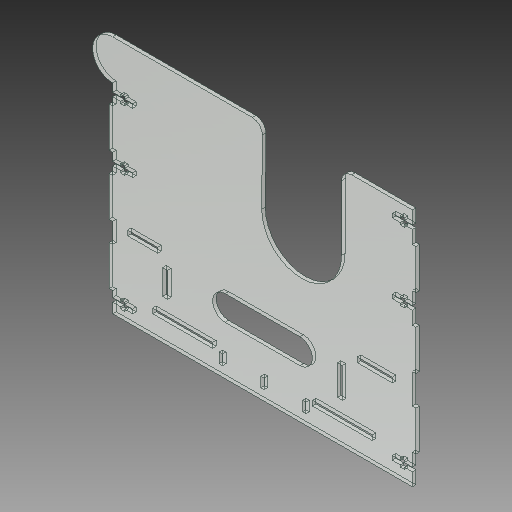
# Autodesk Inventor part: Lat_Der_Caja
Saved by Autodesk Inventor 2019 (Build 230136000, 136)
## iProperties
Created: 2020-04-06
Part Number: Lat_Der_Caja
Material: Generic
Document SubType Name: Modeling
Designer: Jurgen
Density: 1 g/cm^3
Appearance: Clear
Author: Jurgen
Autodesk Inventor part; units mm, degrees
ref_plane "YZ Plane" through (0, 0, 0) normal (1, 0, 0) x (0, 1, 0)
ref_plane "XZ Plane" through (0, 0, 0) normal (0, 1, 0) x (-1, 0, 0)
ref_plane "XY Plane" through (0, 0, 0) normal (0, 0, 1) x (1, 0, 0)
sketch "Sketch1" plane through (0, 0, 0) normal (0, 0, 1) x (1, 0, 0)
  line L0 (0.3285, -0.1681) -> (0.3285, -5.1681)
  line L1 (60.3285, -5.1681) -> (0.3285, -5.1681)
  line L2 (60.3285, -0.1681) -> (60.3285, -5.1681)
  line L3 (0.3285, -0.1681) -> (60.3285, -0.1681)
  line L4 (15.3285, 39.8319) -> (15.3285, 14.8319)
  line L5 (15.3285, 14.8319) -> (10.3285, 14.8319)
  line L6 (10.3285, 14.8319) -> (10.3285, 39.8319)
  line L7 (15.3285, 39.8319) -> (10.3285, 39.8319)
  line L8 (-24.6715, 54.8319) -> (-24.6715, 49.8319)
  line L9 (-24.6715, 54.8319) -> (5.3285, 54.8319)
  line L10 (5.3285, 49.8319) -> (-24.6715, 49.8319)
  line L11 (5.3285, 54.8319) -> (5.3285, 49.8319)
  line L12 (220.3285, -5.1681) -> (160.3285, -5.1681)
  line L13 (160.3285, -0.1681) -> (160.3285, -5.1681)
  line L14 (160.3285, -0.1681) -> (220.3285, -0.1681)
  line L15 (220.3285, -0.1681) -> (220.3285, -5.1681)
  line L16 (190.3285, 14.8319) -> (185.3285, 14.8319)
  line L17 (185.3285, 14.8319) -> (185.3285, 44.8319)
  line L18 (190.3285, 44.8319) -> (190.3285, 14.8319)
  line L19 (190.3285, 44.8319) -> (185.3285, 44.8319)
  line L20 (205.3285, 59.8319) -> (205.3285, 54.8319)
  line L21 (240.3285, 59.8319) -> (205.3285, 59.8319)
  line L22 (240.3285, 54.8319) -> (205.3285, 54.8319)
  line L23 (240.3285, 59.8319) -> (240.3285, 54.8319)
  line L24 (260.3283, -5.1682) -> (260.3283, 214.8318) construction
  line L25 (260.3283, 214.8318) -> (230.3283, 214.8318) construction
  circle A0 centre (149.5, 140) radius 18.5 construction
  circle A1 centre (149.5, 140) radius 12.5 construction
  arc A2 (132.0393, 133.8144) -> (122.7954, 140) centre (122.7954, 130) ccw construction
  arc A3 (134.5683, 127.6856) -> (143.8122, 121.5) centre (143.8122, 131.5) ccw construction
  line L26 (132.0393, 133.8144) -> (134.5683, 127.6856) construction
  line L27 (143.8122, 121.5) -> (185.1878, 121.5) construction
  arc A4 (185.1878, 121.5) -> (194.4317, 127.6856) centre (185.1878, 131.5) ccw construction
  line L28 (194.4317, 127.6856) -> (196.9607, 133.8144) construction
  arc A5 (206.2046, 140) -> (196.9607, 133.8144) centre (206.2046, 130) ccw construction
  line L29 (206.2046, 140) -> (250, 140) construction
  line L30 (81.6779, 140) -> (122.7954, 140) construction
  line L31 (-39.6717, -25.1682) -> (260.3283, -25.1682)
  line L32 (260.3283, -25.1682) -> (260.3283, 214.8318)
  circle A6 centre (149.5, 140) radius 40 construction
  line L33 (-39.6717, 214.8318) -> (-39.6717, -25.1682)
  line L34 (-39.6717, 214.8318) -> (80.3283, 214.8318)
  line L35 (260.3283, 214.8318) -> (-39.6717, 214.8318) construction
  line L36 (215.3283, 214.8318) -> (260.3283, 214.8318) construction
  line L37 (215.3283, 214.8318) -> (260.3283, 214.8318)
  line L38 (109.5, 140) -> (189.5, 140) construction
  arc A7 (109.5, 140) -> (189.5, 140) centre (149.5, 140) ccw
  line L39 (109.5, 140) -> (110.3283, 214.8318)
  line L40 (110.3283, 214.8318) -> (80.3283, 214.8318)
  line L41 (189.5, 140) -> (189.5, 214.8318)
  line L42 (189.5, 214.8318) -> (215.3283, 214.8318)
  line L43 (0.3283, -25.1682) -> (0.3283, 214.8318) construction
  point P0 (0, 0)
  point P1 (113.145, 123.3174)
  point P2 (184.723, 121.0438)
  dimension "d0" = 300
  dimension "d1" = 220
  dimension "d2" = 80
  dimension "d3" = 240
  dimension "d6" = 45
  dimension "d84" = 40
  constraints: 88 end point, 14 point on circle, 8 centre point, 6 horizontal, 5 point on line, 4 vertical, 3 collinear, 2 perpendicular, 1 coincident, 1 concentric, 1 midpoint, 19 other
  measures "d0" distance of L33.start L24.end
  measures "d1" distance of L24.start L24.end
  measures "d2" diameter of A6
  measures "d3" distance of L33.start L31.start
  measures "d6" distance of L24.end L36.start
  measures "d84" distance between parallel lines of L33 L43
extrude "Extrusion1" add sketch "Sketch1" along normal blind 3.5
fillet "Fillet1" radius 10 2 edges at (110.3283, 214.8318, 1.75) (189.5, 214.8318, 1.75)
sketch "Sketch3" plane through (0, 0, 3.5) normal (0, 0, 1) x (1, 0, 0)
  arc A0 (199.5, 214.8318) -> (189.5, 204.8318) centre (199.5, 204.8318) ccw construction
  line L0 (189.5, 204.8318) -> (189.5, 140) construction
  arc A1 (109.5, 140) -> (189.5, 140) centre (149.5, 140) ccw construction
  line L1 (109.5, 140) -> (110.2164, 204.7211) construction
  arc A2 (110.2164, 204.7211) -> (100.217, 214.8318) centre (100.217, 204.8318) ccw construction
  line L2 (100.217, 214.8318) -> (-39.6717, 214.8318) construction
  line L3 (-39.6717, 214.8318) -> (-39.6717, -25.1682) construction
  line L4 (-39.6717, -25.1682) -> (260.3283, -25.1682) construction
  line L5 (260.3283, -25.1682) -> (260.3283, 214.8318) construction
  line L6 (260.3283, 214.8318) -> (199.5, 214.8318) construction
  line L7 (160.3285, -5.1681) -> (160.3285, -0.1681) construction
  line L8 (160.3285, -0.1681) -> (220.3285, -0.1681) construction
  line L9 (220.3285, -0.1681) -> (220.3285, -5.1681) construction
  line L10 (220.3285, -5.1681) -> (160.3285, -5.1681) construction
  line L11 (0.3285, -0.1681) -> (60.3285, -0.1681) construction
  line L12 (60.3285, -0.1681) -> (60.3285, -5.1681) construction
  line L13 (60.3285, -5.1681) -> (0.3285, -5.1681) construction
  line L14 (0.3285, -5.1681) -> (0.3285, -0.1681) construction
  line L15 (205.3285, 59.8319) -> (240.3285, 59.8319) construction
  line L16 (240.3285, 59.8319) -> (240.3285, 54.8319) construction
  line L17 (240.3285, 54.8319) -> (205.3285, 54.8319) construction
  line L18 (205.3285, 54.8319) -> (205.3285, 59.8319) construction
  line L19 (185.3285, 14.8319) -> (185.3285, 44.8319) construction
  line L20 (185.3285, 44.8319) -> (190.3285, 44.8319) construction
  line L21 (190.3285, 44.8319) -> (190.3285, 14.8319) construction
  line L22 (190.3285, 14.8319) -> (185.3285, 14.8319) construction
  line L23 (-24.6715, 54.8319) -> (5.3285, 54.8319) construction
  line L24 (5.3285, 54.8319) -> (5.3285, 49.8319) construction
  line L25 (5.3285, 49.8319) -> (-24.6715, 49.8319) construction
  line L26 (-24.6715, 49.8319) -> (-24.6715, 54.8319) construction
  line L27 (15.3285, 14.8319) -> (10.3285, 14.8319) construction
  line L28 (10.3285, 14.8319) -> (10.3285, 39.8319) construction
  line L29 (10.3285, 39.8319) -> (15.3285, 39.8319) construction
  line L30 (15.3285, 39.8319) -> (15.3285, 14.8319) construction
  line L31 (-39.6717, 214.8318) -> (-39.6717, -25.1682) construction
  arc A3 (-39.6717, 174.8318) -> (-50.6681, 178.1261) centre (-39.6717, 194.8318) ccw construction
  arc A4 (-39.6717, 214.8318) -> (-50.6681, 178.1261) centre (-39.6717, 194.8318) ccw
  line L32 (-39.6717, 174.8318) -> (-39.6717, 159.8318)
  line L33 (-39.6717, 174.8318) -> (-39.6717, 214.8318)
  line L34 (-39.6717, 94.8318) -> (-43.1717, 94.8318)
  line L35 (-43.1717, 94.8318) -> (-43.1717, 54.8318)
  line L36 (-43.1717, 54.8318) -> (-39.6717, 54.8318)
  line L37 (-39.6717, 54.8318) -> (-39.6717, 94.8318)
  line L38 (-39.6717, -5.1682) -> (-43.1717, -5.1682)
  line L39 (-43.1717, -5.1682) -> (-43.1717, 34.8318)
  line L40 (-43.1717, 34.8318) -> (-39.6717, 34.8318)
  line L41 (-39.6717, 34.8318) -> (-39.6717, -5.1682)
  line L42 (-39.6717, 154.8318) -> (-43.1717, 154.8318)
  line L43 (-43.1717, 154.8318) -> (-43.1717, 114.8318)
  line L44 (-43.1717, 114.8318) -> (-39.6717, 114.8318)
  line L45 (-39.6717, 114.8318) -> (-39.6717, 154.8318)
  line L46 (-39.6717, -25.1682) -> (-39.6717, 214.8318) construction
  line L47 (110.3283, -25.1682) -> (110.3283, 54.8318) construction
  line L48 (260.3283, 184.8318) -> (263.8283, 184.8318)
  line L49 (263.8283, 184.8318) -> (263.8283, 144.8318)
  line L50 (263.8283, 144.8318) -> (260.3283, 144.8318)
  line L51 (260.3283, 144.8318) -> (260.3283, 184.8318)
  line L52 (260.3283, -25.1682) -> (260.3283, 214.8318) construction
  line L53 (260.3283, 114.8318) -> (263.8283, 114.8318)
  line L54 (263.8283, 114.8318) -> (263.8283, 74.8318)
  line L55 (263.8283, 74.8318) -> (260.3283, 74.8318)
  line L56 (260.3283, 74.8318) -> (260.3283, 114.8318)
  line L57 (260.3283, 44.8318) -> (263.8283, 44.8318)
  line L58 (263.8283, 44.8318) -> (263.8283, 4.8318)
  line L59 (263.8283, 4.8318) -> (260.3283, 4.8318)
  line L60 (260.3283, 4.8318) -> (260.3283, 44.8318)
  arc A5 (-39.6717, 214.8318) -> (-39.6717, 174.8318) centre (-39.6717, 194.8318) ccw
  point P0 (0, 0)
  dimension "d21" = 40
  dimension "d22" = 20
  dimension "d23" = 15
  dimension "d24" = 3.5
  dimension "d25" = 40
  dimension "d26" = 3.5
  dimension "d27" = 40
  dimension "d28" = 20
  dimension "d29" = 20
  dimension "d30" = 3.5
  dimension "d31" = 40
  dimension "d32" = 20
  dimension "d35" = 3.5
  dimension "d36" = 40
  dimension "d37" = 3.5
  dimension "d38" = 40
  dimension "d39" = 3.5
  dimension "d40" = 40
  dimension "d41" = 30
  dimension "d42" = 30
  dimension "d43" = 30
  constraints: 56 end point, 12 parallel, 8 point on line, 6 horizontal, 6 perpendicular, 6 point on circle, 3 centre point, 3 tangent, 1 midpoint, 1 vertical
  measures "d21" diameter of A3
  measures "d22" distance from line of L2 A3.centre
  measures "d23" distance of L32.start L32.end
  measures "d24" distance of L36.end L35.end
  measures "d25" distance of L35.end L34.end
  measures "d26" distance of L39.end L40.end
  measures "d27" distance of L38.end L39.end
  measures "d28" distance between parallel lines of L4 L38
  measures "d29" distance between parallel lines of L40 L36
  measures "d30" distance of L44.end L43.end
  measures "d31" distance of L43.end L42.end
  measures "d32" distance from line of L34.end L44
  measures "d35" distance of L49.end L50.end
  measures "d36" distance of L48.end L49.end
  measures "d37" distance of L54.end L55.end
  measures "d38" distance of L53.end L54.end
  measures "d39" distance of L58.end L59.end
  measures "d40" distance of L57.end L58.end
  measures "d41" distance between parallel lines of L4 L59
  measures "d42" distance between parallel lines of L57 L55
  measures "d43" distance between parallel lines of L53 L50
extrude "Extrusion3" add sketch "Sketch3" against normal blind 3.5
sketch "Sketch4" plane through (0, 0, 3.5) normal (0, 0, 1) x (1, 0, 0)
  arc A0 (199.5, 214.8318) -> (189.5, 204.8318) centre (199.5, 204.8318) ccw construction
  line L0 (189.5, 204.8318) -> (189.5, 140) construction
  arc A1 (109.5, 140) -> (189.5, 140) centre (149.5, 140) ccw construction
  line L1 (109.5, 140) -> (110.2164, 204.7211) construction
  arc A2 (110.2164, 204.7211) -> (100.217, 214.8318) centre (100.217, 204.8318) ccw construction
  line L2 (100.217, 214.8318) -> (-39.6717, 214.8318) construction
  arc A3 (-39.6717, 214.8318) -> (-39.6717, 174.8318) centre (-39.6717, 194.8318) ccw construction
  line L3 (-39.6717, 174.8318) -> (-39.6717, 154.8318) construction
  line L4 (-39.6717, 154.8318) -> (-43.1717, 154.8318) construction
  line L5 (-43.1717, 154.8318) -> (-43.1717, 114.8318) construction
  line L6 (-43.1717, 114.8318) -> (-39.6717, 114.8318) construction
  line L7 (-39.6717, 114.8318) -> (-39.6717, 94.8318) construction
  line L8 (-39.6717, 94.8318) -> (-43.1717, 94.8318) construction
  line L9 (-43.1717, 94.8318) -> (-43.1717, 54.8318) construction
  line L10 (-43.1717, 54.8318) -> (-39.6717, 54.8318) construction
  line L11 (-39.6717, 54.8318) -> (-39.6717, 34.8318) construction
  line L12 (-43.1717, 34.8318) -> (-39.6717, 34.8318) construction
  line L13 (-43.1717, -5.1682) -> (-43.1717, 34.8318) construction
  line L14 (-39.6717, -5.1682) -> (-43.1717, -5.1682) construction
  line L15 (-39.6717, -5.1682) -> (-39.6717, -25.1682) construction
  line L16 (-39.6717, -25.1682) -> (260.3283, -25.1682) construction
  line L17 (260.3283, -25.1682) -> (260.3283, 4.8318) construction
  line L18 (263.8283, 4.8318) -> (260.3283, 4.8318) construction
  line L19 (263.8283, 44.8318) -> (263.8283, 4.8318) construction
  line L20 (260.3283, 44.8318) -> (263.8283, 44.8318) construction
  line L21 (260.3283, 44.8318) -> (260.3283, 74.8318) construction
  line L22 (263.8283, 74.8318) -> (260.3283, 74.8318) construction
  line L23 (263.8283, 114.8318) -> (263.8283, 74.8318) construction
  line L24 (260.3283, 114.8318) -> (263.8283, 114.8318) construction
  line L25 (260.3283, 114.8318) -> (260.3283, 144.8318) construction
  line L26 (263.8283, 144.8318) -> (260.3283, 144.8318) construction
  line L27 (263.8283, 184.8318) -> (263.8283, 144.8318) construction
  line L28 (260.3283, 184.8318) -> (263.8283, 184.8318) construction
  line L29 (260.3283, 184.8318) -> (260.3283, 214.8318) construction
  line L30 (260.3283, 214.8318) -> (199.5, 214.8318) construction
  line L31 (160.3285, -5.1681) -> (160.3285, -0.1681) construction
  line L32 (160.3285, -0.1681) -> (220.3285, -0.1681) construction
  line L33 (220.3285, -0.1681) -> (220.3285, -5.1681) construction
  line L34 (220.3285, -5.1681) -> (160.3285, -5.1681) construction
  line L35 (0.3285, -0.1681) -> (60.3285, -0.1681) construction
  line L36 (60.3285, -0.1681) -> (60.3285, -5.1681) construction
  line L37 (60.3285, -5.1681) -> (0.3285, -5.1681) construction
  line L38 (0.3285, -5.1681) -> (0.3285, -0.1681) construction
  line L39 (205.3285, 59.8319) -> (240.3285, 59.8319) construction
  line L40 (240.3285, 59.8319) -> (240.3285, 54.8319) construction
  line L41 (240.3285, 54.8319) -> (205.3285, 54.8319) construction
  line L42 (205.3285, 54.8319) -> (205.3285, 59.8319) construction
  line L43 (185.3285, 14.8319) -> (185.3285, 44.8319) construction
  line L44 (185.3285, 44.8319) -> (190.3285, 44.8319) construction
  line L45 (190.3285, 44.8319) -> (190.3285, 14.8319) construction
  line L46 (190.3285, 14.8319) -> (185.3285, 14.8319) construction
  line L47 (-24.6715, 54.8319) -> (5.3285, 54.8319) construction
  line L48 (5.3285, 54.8319) -> (5.3285, 49.8319) construction
  line L49 (5.3285, 49.8319) -> (-24.6715, 49.8319) construction
  line L50 (-24.6715, 49.8319) -> (-24.6715, 54.8319) construction
  line L51 (15.3285, 14.8319) -> (10.3285, 14.8319) construction
  line L52 (10.3285, 14.8319) -> (10.3285, 39.8319) construction
  line L53 (10.3285, 39.8319) -> (15.3285, 39.8319) construction
  line L54 (15.3285, 39.8319) -> (15.3285, 14.8319) construction
  line L55 (-39.6717, 174.8318) -> (-39.6717, 154.8318) construction
  line L56 (-39.6717, 162.8318) -> (-19.6717, 162.8318) construction
  line L57 (-19.6717, 162.8318) -> (-19.6717, 166.8318) construction
  line L58 (-19.6717, 166.8318) -> (-39.6717, 166.8318) construction
  line L59 (-39.6717, 166.8318) -> (-39.6717, 162.8318) construction
  line L60 (-39.6717, 164.8318) -> (-19.6717, 164.8318) construction
  line L61 (-31.6717, 160.8318) -> (-27.6717, 160.8318) construction
  line L62 (-27.6717, 160.8318) -> (-27.6717, 168.8318) construction
  line L63 (-27.6717, 168.8318) -> (-31.6717, 168.8318) construction
  line L64 (-31.6717, 168.8318) -> (-31.6717, 160.8318) construction
  line L65 (-31.6717, 160.8318) -> (-27.6717, 168.8318) construction
  line L66 (-27.6717, 160.8318) -> (-31.6717, 168.8318) construction
  line L67 (-39.6717, 166.8318) -> (-39.6717, 162.8318)
  line L68 (-39.6717, 162.8318) -> (-31.6717, 162.8318)
  line L69 (-31.6717, 162.8318) -> (-31.6717, 160.8318)
  line L70 (-31.6717, 160.8318) -> (-27.6717, 160.8318)
  line L71 (-27.6717, 160.8318) -> (-27.6717, 162.8318)
  line L72 (-27.6717, 162.8318) -> (-19.6717, 162.8318)
  line L73 (-19.6717, 162.8318) -> (-19.6717, 166.8318)
  line L74 (-19.6717, 166.8318) -> (-27.6717, 166.8318)
  line L75 (-27.6717, 166.8318) -> (-27.6717, 168.8318)
  line L76 (-27.6717, 168.8318) -> (-31.6717, 168.8318)
  line L77 (-31.6717, 168.8318) -> (-31.6717, 166.8318)
  line L78 (-31.6717, 166.8318) -> (-39.6717, 166.8318)
  line L79 (-39.6717, 102.8318) -> (-19.6717, 102.8318) construction
  line L80 (-19.6717, 102.8318) -> (-19.6717, 106.8318) construction
  line L81 (-19.6717, 106.8318) -> (-39.6717, 106.8318) construction
  line L82 (-39.6717, 106.8318) -> (-39.6717, 102.8318) construction
  line L83 (-39.6717, 104.8318) -> (-19.6717, 104.8318) construction
  line L84 (-31.6717, 100.8318) -> (-27.6717, 100.8318) construction
  line L85 (-27.6717, 100.8318) -> (-27.6717, 108.8318) construction
  line L86 (-27.6717, 108.8318) -> (-31.6717, 108.8318) construction
  line L87 (-31.6717, 108.8318) -> (-31.6717, 100.8318) construction
  line L88 (-31.6717, 100.8318) -> (-27.6717, 108.8318) construction
  line L89 (-27.6717, 100.8318) -> (-31.6717, 108.8318) construction
  line L90 (-39.6717, 106.8318) -> (-39.6717, 102.8318)
  line L91 (-39.6717, 102.8318) -> (-31.6717, 102.8318)
  line L92 (-31.6717, 102.8318) -> (-31.6717, 100.8318)
  line L93 (-31.6717, 100.8318) -> (-27.6717, 100.8318)
  line L94 (-27.6717, 100.8318) -> (-27.6717, 102.8318)
  line L95 (-27.6717, 102.8318) -> (-19.6717, 102.8318)
  line L96 (-19.6717, 102.8318) -> (-19.6717, 106.8318)
  line L97 (-19.6717, 106.8318) -> (-27.6717, 106.8318)
  line L98 (-27.6717, 106.8318) -> (-27.6717, 108.8318)
  line L99 (-27.6717, 108.8318) -> (-31.6717, 108.8318)
  line L100 (-31.6717, 108.8318) -> (-31.6717, 106.8318)
  line L101 (-31.6717, 106.8318) -> (-39.6717, 106.8318)
  line L102 (-39.6717, -15.1682) -> (-19.6717, -15.1682) construction
  line L103 (-19.6717, -15.1682) -> (-19.6717, -11.1682) construction
  line L104 (-19.6717, -11.1682) -> (-39.6717, -11.1682) construction
  line L105 (-39.6717, -11.1682) -> (-39.6717, -15.1682) construction
  line L106 (-39.6717, -13.1682) -> (-19.6717, -13.1682) construction
  line L107 (-31.6717, -17.1682) -> (-27.6717, -17.1682) construction
  line L108 (-27.6717, -17.1682) -> (-27.6717, -9.1682) construction
  line L109 (-27.6717, -9.1682) -> (-31.6717, -9.1682) construction
  line L110 (-31.6717, -9.1682) -> (-31.6717, -17.1682) construction
  line L111 (-31.6717, -17.1682) -> (-27.6717, -9.1682) construction
  line L112 (-27.6717, -17.1682) -> (-31.6717, -9.1682) construction
  line L113 (-39.6717, -11.1682) -> (-39.6717, -15.1682)
  line L114 (-39.6717, -15.1682) -> (-31.6717, -15.1682)
  line L115 (-31.6717, -15.1682) -> (-31.6717, -17.1682)
  line L116 (-31.6717, -17.1682) -> (-27.6717, -17.1682)
  line L117 (-27.6717, -17.1682) -> (-27.6717, -15.1682)
  line L118 (-27.6717, -15.1682) -> (-19.6717, -15.1682)
  line L119 (-19.6717, -15.1682) -> (-19.6717, -11.1682)
  line L120 (-19.6717, -11.1682) -> (-27.6717, -11.1682)
  line L121 (-27.6717, -11.1682) -> (-27.6717, -9.1682)
  line L122 (-27.6717, -9.1682) -> (-31.6717, -9.1682)
  line L123 (-31.6717, -9.1682) -> (-31.6717, -11.1682)
  line L124 (-31.6717, -11.1682) -> (-39.6717, -11.1682)
  line L125 (260.3283, 214.8318) -> (199.5, 214.8318) construction
  line L126 (-39.6717, -25.1682) -> (260.3283, -25.1682) construction
  line L127 (260.3283, -25.1682) -> (260.3283, 214.8318) construction
  line L128 (260.3283, 214.8318) -> (-39.6717, 214.8318) construction
  line L129 (-39.6717, 214.8318) -> (-39.6717, -25.1682) construction
  line L130 (110.3283, -25.1682) -> (110.3283, 56.8318) construction
  line L131 (263.8283, 114.8318) -> (260.3283, 114.8318) construction
  line L132 (260.3283, 114.8318) -> (260.3283, 94.8318) construction
  line L133 (240.3283, 197.8318) -> (240.3283, 201.8318) construction
  line L134 (240.3283, 197.8318) -> (240.3283, 201.8318)
  line L135 (248.3283, 197.8318) -> (240.3283, 197.8318)
  line L136 (260.3283, 197.8318) -> (240.3283, 197.8318) construction
  line L137 (240.3283, 201.8318) -> (248.3283, 201.8318)
  line L138 (240.3283, 201.8318) -> (260.3283, 201.8318) construction
  line L139 (260.3283, 199.8318) -> (240.3283, 199.8318) construction
  line L140 (248.3283, 201.8318) -> (248.3283, 203.8318)
  line L141 (248.3283, 195.8318) -> (248.3283, 197.8318)
  line L142 (252.3283, 195.8318) -> (248.3283, 195.8318)
  line L143 (260.3283, 197.8318) -> (252.3283, 197.8318)
  line L144 (252.3283, 197.8318) -> (252.3283, 195.8318)
  line L145 (252.3283, 201.8318) -> (260.3283, 201.8318)
  line L146 (252.3283, 203.8318) -> (252.3283, 201.8318)
  line L147 (248.3283, 203.8318) -> (252.3283, 203.8318)
  line L148 (252.3283, 195.8318) -> (248.3283, 195.8318) construction
  line L149 (260.3283, 201.8318) -> (260.3283, 197.8318) construction
  line L150 (260.3283, 201.8318) -> (260.3283, 197.8318)
  line L151 (248.3283, 195.8318) -> (248.3283, 203.8318) construction
  line L152 (248.3283, 203.8318) -> (252.3283, 203.8318) construction
  line L153 (252.3283, 195.8318) -> (248.3283, 203.8318) construction
  line L154 (248.3283, 195.8318) -> (252.3283, 203.8318) construction
  line L155 (252.3283, 203.8318) -> (252.3283, 195.8318) construction
  line L156 (252.3283, 125.8318) -> (248.3283, 125.8318)
  line L157 (240.3283, 127.8318) -> (240.3283, 131.8318) construction
  line L158 (260.3283, 127.8318) -> (252.3283, 127.8318)
  line L159 (252.3283, 131.8318) -> (260.3283, 131.8318)
  line L160 (260.3283, 131.8318) -> (260.3283, 127.8318) construction
  line L161 (260.3283, 131.8318) -> (260.3283, 127.8318)
  line L162 (240.3283, 127.8318) -> (240.3283, 131.8318)
  line L163 (248.3283, 127.8318) -> (240.3283, 127.8318)
  line L164 (240.3283, 131.8318) -> (248.3283, 131.8318)
  line L165 (260.3283, 127.8318) -> (240.3283, 127.8318) construction
  line L166 (240.3283, 131.8318) -> (260.3283, 131.8318) construction
  line L167 (260.3283, 129.8318) -> (240.3283, 129.8318) construction
  line L168 (252.3283, 125.8318) -> (248.3283, 125.8318) construction
  line L169 (248.3283, 125.8318) -> (248.3283, 127.8318)
  line L170 (252.3283, 127.8318) -> (252.3283, 125.8318)
  line L171 (248.3283, 131.8318) -> (248.3283, 133.8318)
  line L172 (252.3283, 133.8318) -> (252.3283, 131.8318)
  line L173 (248.3283, 133.8318) -> (252.3283, 133.8318)
  line L174 (248.3283, 133.8318) -> (252.3283, 133.8318) construction
  line L175 (248.3283, 125.8318) -> (248.3283, 133.8318) construction
  line L176 (248.3283, 125.8318) -> (252.3283, 133.8318) construction
  line L177 (252.3283, 125.8318) -> (248.3283, 133.8318) construction
  line L178 (252.3283, 133.8318) -> (252.3283, 125.8318) construction
  line L179 (252.3283, -14.1682) -> (248.3283, -14.1682)
  line L180 (240.3283, -12.1682) -> (240.3283, -8.1682) construction
  line L181 (260.3283, -12.1682) -> (252.3283, -12.1682)
  line L182 (252.3283, -8.1682) -> (260.3283, -8.1682)
  line L183 (260.3283, -8.1682) -> (260.3283, -12.1682) construction
  line L184 (260.3283, -8.1682) -> (260.3283, -12.1682)
  line L185 (240.3283, -12.1682) -> (240.3283, -8.1682)
  line L186 (248.3283, -12.1682) -> (240.3283, -12.1682)
  line L187 (240.3283, -8.1682) -> (248.3283, -8.1682)
  line L188 (260.3283, -12.1682) -> (240.3283, -12.1682) construction
  line L189 (240.3283, -8.1682) -> (260.3283, -8.1682) construction
  line L190 (260.3283, -10.1682) -> (240.3283, -10.1682) construction
  line L191 (252.3283, -14.1682) -> (248.3283, -14.1682) construction
  line L192 (248.3283, -14.1682) -> (248.3283, -12.1682)
  line L193 (252.3283, -12.1682) -> (252.3283, -14.1682)
  line L194 (248.3283, -8.1682) -> (248.3283, -6.1682)
  line L195 (252.3283, -6.1682) -> (252.3283, -8.1682)
  line L196 (248.3283, -6.1682) -> (252.3283, -6.1682)
  line L197 (248.3283, -6.1682) -> (252.3283, -6.1682) construction
  line L198 (248.3283, -14.1682) -> (248.3283, -6.1682) construction
  line L199 (248.3283, -14.1682) -> (252.3283, -6.1682) construction
  line L200 (252.3283, -14.1682) -> (248.3283, -6.1682) construction
  line L201 (252.3283, -6.1682) -> (252.3283, -14.1682) construction
  point P0 (0, 0)
  point P1 (-29.6717, 164.8318)
  point P2 (-29.6717, 104.8318)
  point P3 (-29.6717, -13.1682)
  point P4 (250.3283, 199.8318)
  point P5 (250.3283, 129.8318)
  point P6 (250.3283, -10.1682)
  dimension "d46" = 20
  dimension "d47" = 4
  dimension "d48" = 4
  dimension "d49" = 8
  dimension "d50" = 8
  dimension "d51" = 8
  dimension "d52" = 20
  dimension "d53" = 4
  dimension "d54" = 4
  dimension "d55" = 8
  dimension "d56" = 8
  dimension "d57" = 20
  dimension "d58" = 4
  dimension "d59" = 4
  dimension "d60" = 8
  dimension "d61" = 8
  dimension "d62" = 8
  dimension "d63" = 6
  dimension "d65" = 20
  dimension "d66" = 8
  dimension "d67" = 4
  dimension "d68" = 8
  dimension "d69" = 13
  dimension "d70" = 2
  dimension "d71" = 8
  dimension "d72" = 4
  dimension "d73" = 2
  dimension "d74" = 8
  dimension "d75" = 4
  dimension "d76" = 2
  dimension "d77" = 13
  dimension "d78" = 13
  dimension "d79" = 8
  dimension "d80" = 8
  constraints: 290 end point, 49 point on line, 25 midpoint, 23 perpendicular, 14 parallel, 7 horizontal, 3 collinear, 3 vertical, 1 symmetric about line
  measures "d46" distance of L58.end L57.end
  measures "d47" distance of L57.end L56.end
  measures "d48" distance of L63.end L62.end
  measures "d49" distance of L62.end L61.end
  measures "d50" distance between parallel lines of L57 L62
  measures "d51" distance between parallel lines of L4 L68
  measures "d52" distance of L81.end L81.start
  measures "d53" distance of L81.start L79.end
  measures "d54" distance of L86.end L86.start
  measures "d55" distance of L86.start L84.end
  measures "d56" distance between parallel lines of L80 L85
  measures "d57" distance of L104.end L104.start
  measures "d58" distance of L104.start L102.end
  measures "d59" distance of L109.end L109.start
  measures "d60" distance of L109.start L107.end
  measures "d61" distance between parallel lines of L103 L108
  measures "d62" distance between parallel lines of L8 L79
  measures "d63" distance between parallel lines of L14 L124
  measures "d65" distance between parallel lines of L29 L133
  measures "d66" distance between parallel lines of L142 L152
  measures "d67" distance between parallel lines of L135 L137
  measures "d68" distance between parallel lines of L29 L155
  measures "d69" distance between parallel lines of L28 L143
  measures "d70" distance between parallel lines of L135 L142
  measures "d71" distance between parallel lines of L156 L174
  measures "d72" distance between parallel lines of L163 L164
  measures "d73" distance between parallel lines of L163 L156
  measures "d74" distance between parallel lines of L179 L197
  measures "d75" distance between parallel lines of L186 L187
  measures "d76" distance between parallel lines of L186 L179
  measures "d77" distance between parallel lines of L26 L159
  measures "d78" distance between parallel lines of L18 L189
  measures "d79" distance between parallel lines of L25 L178
  measures "d80" distance between parallel lines of L127 L193
extrude "Extrusion4" cut sketch "Sketch4" against normal blind 3.5
sketch "Sketch5" plane through (0, 0, 0) normal (0, 0, -1) x (-1, 0, 0)
  line L0 (-66.8283, -15.1682) -> (-70.3283, -15.1682)
  line L1 (-70.3283, -15.1682) -> (-70.3283, -5.1682)
  line L2 (-70.3283, -5.1682) -> (-66.8283, -5.1682)
  line L3 (-66.8283, -5.1682) -> (-66.8283, -15.1682)
  line L4 (-150.3283, -15.1682) -> (-153.8283, -15.1682)
  line L5 (-153.8283, -15.1682) -> (-153.8283, -5.1682)
  line L6 (-153.8283, -5.1682) -> (-150.3283, -5.1682)
  line L7 (-150.3283, -5.1682) -> (-150.3283, -15.1682)
  line L8 (-108.5783, -15.1682) -> (-112.0783, -15.1682)
  line L9 (-112.0783, -15.1682) -> (-112.0783, -5.1682)
  line L10 (-112.0783, -5.1682) -> (-108.5783, -5.1682)
  line L11 (-108.5783, -5.1682) -> (-108.5783, -15.1682)
  arc A0 (-72.8283, 23.5818) -> (-72.8283, 48.5818) centre (-72.8283, 36.0818) ccw
  line L12 (-72.8283, 23.5818) -> (-147.8283, 23.5818)
  arc A1 (-147.8283, 48.5818) -> (-147.8283, 23.5818) centre (-147.8283, 36.0818) ccw
  line L13 (-147.8283, 48.5818) -> (-72.8283, 48.5818)
  line L14 (-15.3283, 39.8318) -> (-10.3283, 39.8318) construction
  line L15 (-10.3283, 39.8318) -> (-10.3283, 14.8318) construction
  line L16 (-10.3283, 14.8318) -> (-15.3283, 14.8318) construction
  line L17 (-15.3283, 14.8318) -> (-15.3283, 39.8318) construction
  line L18 (-190.3283, 44.8318) -> (-185.3283, 44.8318) construction
  line L19 (-185.3283, 44.8318) -> (-185.3283, 14.8318) construction
  line L20 (-185.3283, 14.8318) -> (-190.3283, 14.8318) construction
  line L21 (-190.3283, 14.8318) -> (-190.3283, 44.8318) construction
  line L22 (-5.3283, 49.8318) -> (-5.3283, 54.8318) construction
  line L23 (-5.3283, 54.8318) -> (24.6717, 54.8318) construction
  line L24 (24.6717, 54.8318) -> (24.6717, 49.8318) construction
  line L25 (24.6717, 49.8318) -> (-5.3283, 49.8318) construction
  line L26 (-205.3283, 59.8318) -> (-205.3283, 54.8318) construction
  line L27 (-205.3283, 54.8318) -> (-240.3283, 54.8318) construction
  line L28 (-240.3283, 54.8318) -> (-240.3283, 59.8318) construction
  line L29 (-240.3283, 59.8318) -> (-205.3283, 59.8318) construction
  line L30 (-160.3283, -0.1682) -> (-160.3283, -5.1682) construction
  line L31 (-160.3283, -5.1682) -> (-220.3283, -5.1682) construction
  line L32 (-220.3283, -5.1682) -> (-220.3283, -0.1682) construction
  line L33 (-220.3283, -0.1682) -> (-160.3283, -0.1682) construction
  line L34 (-0.3283, -0.1682) -> (-0.3283, -5.1682) construction
  line L35 (-0.3283, -5.1682) -> (-60.3283, -5.1682) construction
  line L36 (-60.3283, -5.1682) -> (-60.3283, -0.1682) construction
  line L37 (-60.3283, -0.1682) -> (-0.3283, -0.1682) construction
  line L38 (-260.3283, 131.8318) -> (-252.3283, 131.8318) construction
  line L39 (-252.3283, 131.8318) -> (-252.3283, 133.8318) construction
  line L40 (-252.3283, 133.8318) -> (-248.3283, 133.8318) construction
  line L41 (-248.3283, 133.8318) -> (-248.3283, 131.8318) construction
  line L42 (-248.3283, 131.8318) -> (-240.3283, 131.8318) construction
  line L43 (-240.3283, 131.8318) -> (-240.3283, 127.8318) construction
  line L44 (-240.3283, 127.8318) -> (-248.3283, 127.8318) construction
  line L45 (-248.3283, 127.8318) -> (-248.3283, 125.8318) construction
  line L46 (-248.3283, 125.8318) -> (-252.3283, 125.8318) construction
  line L47 (-252.3283, 125.8318) -> (-252.3283, 127.8318) construction
  line L48 (-252.3283, 127.8318) -> (-260.3283, 127.8318) construction
  line L49 (-260.3283, 127.8318) -> (-260.3283, 114.8318) construction
  line L50 (-260.3283, 114.8318) -> (-263.8283, 114.8318) construction
  line L51 (-263.8283, 114.8318) -> (-263.8283, 74.8318) construction
  line L52 (-263.8283, 74.8318) -> (-260.3283, 74.8318) construction
  line L53 (-260.3283, 74.8318) -> (-260.3283, 44.8318) construction
  line L54 (-260.3283, 44.8318) -> (-263.8283, 44.8318) construction
  line L55 (-263.8283, 44.8318) -> (-263.8283, 4.8318) construction
  line L56 (-263.8283, 4.8318) -> (-260.3283, 4.8318) construction
  line L57 (-260.3283, 4.8318) -> (-260.3283, -8.1682) construction
  line L58 (-260.3283, -8.1682) -> (-252.3283, -8.1682) construction
  line L59 (-252.3283, -8.1682) -> (-252.3283, -6.1682) construction
  line L60 (-252.3283, -6.1682) -> (-248.3283, -6.1682) construction
  line L61 (-248.3283, -6.1682) -> (-248.3283, -8.1682) construction
  line L62 (-248.3283, -8.1682) -> (-240.3283, -8.1682) construction
  line L63 (-240.3283, -8.1682) -> (-240.3283, -12.1682) construction
  line L64 (-240.3283, -12.1682) -> (-248.3283, -12.1682) construction
  line L65 (-248.3283, -12.1682) -> (-248.3283, -14.1682) construction
  line L66 (-248.3283, -14.1682) -> (-252.3283, -14.1682) construction
  line L67 (-252.3283, -14.1682) -> (-252.3283, -12.1682) construction
  line L68 (-252.3283, -12.1682) -> (-260.3283, -12.1682) construction
  line L69 (-260.3283, -12.1682) -> (-260.3283, -25.1682) construction
  line L70 (-260.3283, -25.1682) -> (39.6717, -25.1682) construction
  line L71 (39.6717, -25.1682) -> (39.6717, -15.1682) construction
  line L72 (39.6717, -15.1682) -> (31.6717, -15.1682) construction
  line L73 (31.6717, -15.1682) -> (31.6717, -17.1682) construction
  line L74 (31.6717, -17.1682) -> (27.6717, -17.1682) construction
  line L75 (27.6717, -17.1682) -> (27.6717, -15.1682) construction
  line L76 (27.6717, -15.1682) -> (19.6717, -15.1682) construction
  line L77 (19.6717, -15.1682) -> (19.6717, -11.1682) construction
  line L78 (19.6717, -11.1682) -> (27.6717, -11.1682) construction
  line L79 (27.6717, -11.1682) -> (27.6717, -9.1682) construction
  line L80 (27.6717, -9.1682) -> (31.6717, -9.1682) construction
  line L81 (31.6717, -9.1682) -> (31.6717, -11.1682) construction
  line L82 (31.6717, -11.1682) -> (39.6717, -11.1682) construction
  line L83 (39.6717, -11.1682) -> (39.6717, -5.1682) construction
  line L84 (39.6717, -5.1682) -> (43.1717, -5.1682) construction
  line L85 (43.1717, -5.1682) -> (43.1717, 34.8318) construction
  line L86 (43.1717, 34.8318) -> (39.6717, 34.8318) construction
  line L87 (39.6717, 34.8318) -> (39.6717, 54.8318) construction
  line L88 (39.6717, 54.8318) -> (43.1717, 54.8318) construction
  line L89 (43.1717, 54.8318) -> (43.1717, 94.8318) construction
  line L90 (43.1717, 94.8318) -> (39.6717, 94.8318) construction
  line L91 (39.6717, 94.8318) -> (39.6717, 102.8318) construction
  line L92 (39.6717, 102.8318) -> (31.6717, 102.8318) construction
  line L93 (31.6717, 102.8318) -> (31.6717, 100.8318) construction
  line L94 (31.6717, 100.8318) -> (27.6717, 100.8318) construction
  line L95 (27.6717, 100.8318) -> (27.6717, 102.8318) construction
  line L96 (27.6717, 102.8318) -> (19.6717, 102.8318) construction
  line L97 (19.6717, 102.8318) -> (19.6717, 106.8318) construction
  line L98 (19.6717, 106.8318) -> (27.6717, 106.8318) construction
  line L99 (27.6717, 106.8318) -> (27.6717, 108.8318) construction
  line L100 (27.6717, 108.8318) -> (31.6717, 108.8318) construction
  line L101 (31.6717, 108.8318) -> (31.6717, 106.8318) construction
  line L102 (31.6717, 106.8318) -> (39.6717, 106.8318) construction
  line L103 (39.6717, 106.8318) -> (39.6717, 114.8318) construction
  line L104 (39.6717, 114.8318) -> (43.1717, 114.8318) construction
  line L105 (43.1717, 114.8318) -> (43.1717, 154.8318) construction
  line L106 (43.1717, 154.8318) -> (39.6717, 154.8318) construction
  line L107 (39.6717, 154.8318) -> (39.6717, 162.8318) construction
  line L108 (39.6717, 162.8318) -> (31.6717, 162.8318) construction
  line L109 (31.6717, 162.8318) -> (31.6717, 160.8318) construction
  line L110 (31.6717, 160.8318) -> (27.6717, 160.8318) construction
  line L111 (27.6717, 160.8318) -> (27.6717, 162.8318) construction
  line L112 (27.6717, 162.8318) -> (19.6717, 162.8318) construction
  line L113 (19.6717, 162.8318) -> (19.6717, 166.8318) construction
  line L114 (19.6717, 166.8318) -> (27.6717, 166.8318) construction
  line L115 (27.6717, 166.8318) -> (27.6717, 168.8318) construction
  line L116 (27.6717, 168.8318) -> (31.6717, 168.8318) construction
  line L117 (31.6717, 168.8318) -> (31.6717, 166.8318) construction
  line L118 (31.6717, 166.8318) -> (39.6717, 166.8318) construction
  line L119 (39.6717, 166.8318) -> (39.6717, 174.8318) construction
  arc A2 (39.6717, 174.8318) -> (39.6717, 214.8318) centre (39.6717, 194.8318) ccw construction
  line L120 (39.6717, 214.8318) -> (-89.8283, 214.8318) construction
  arc A3 (-89.8283, 214.8318) -> (-99.8283, 204.8318) centre (-89.8283, 204.8318) ccw construction
  line L121 (-99.8283, 204.8318) -> (-99.8283, 139.8318) construction
  arc A4 (-199.8283, 139.8318) -> (-99.8283, 139.8318) centre (-149.8283, 139.8318) ccw construction
  line L122 (-199.8283, 139.8318) -> (-199.8283, 204.8318) construction
  arc A5 (-199.8283, 204.8318) -> (-209.8283, 214.8318) centre (-209.8283, 204.8318) ccw construction
  line L123 (-209.8283, 214.8318) -> (-260.3283, 214.8318) construction
  line L124 (-260.3283, 214.8318) -> (-260.3283, 201.8318) construction
  line L125 (-260.3283, 201.8318) -> (-252.3283, 201.8318) construction
  line L126 (-252.3283, 201.8318) -> (-252.3283, 203.8318) construction
  line L127 (-252.3283, 203.8318) -> (-248.3283, 203.8318) construction
  line L128 (-248.3283, 203.8318) -> (-248.3283, 201.8318) construction
  line L129 (-248.3283, 201.8318) -> (-240.3283, 201.8318) construction
  line L130 (-240.3283, 201.8318) -> (-240.3283, 197.8318) construction
  line L131 (-240.3283, 197.8318) -> (-248.3283, 197.8318) construction
  line L132 (-248.3283, 197.8318) -> (-248.3283, 195.8318) construction
  line L133 (-248.3283, 195.8318) -> (-252.3283, 195.8318) construction
  line L134 (-252.3283, 195.8318) -> (-252.3283, 197.8318) construction
  line L135 (-252.3283, 197.8318) -> (-260.3283, 197.8318) construction
  line L136 (-260.3283, 197.8318) -> (-260.3283, 184.8318) construction
  line L137 (-260.3283, 184.8318) -> (-263.8283, 184.8318) construction
  line L138 (-263.8283, 184.8318) -> (-263.8283, 144.8318) construction
  line L139 (-263.8283, 144.8318) -> (-260.3283, 144.8318) construction
  line L140 (-260.3283, 144.8318) -> (-260.3283, 131.8318) construction
  line L141 (39.6717, -25.1682) -> (-260.3283, -25.1682) construction
  point P0 (0, 0)
  point P1 (-110.3283, 97.3318)
  constraints: 282 end point, 12 point on circle, 6 centre point
extrude "Extrusion5" cut sketch "Sketch5" against normal blind 3.5
body "Solid1"
